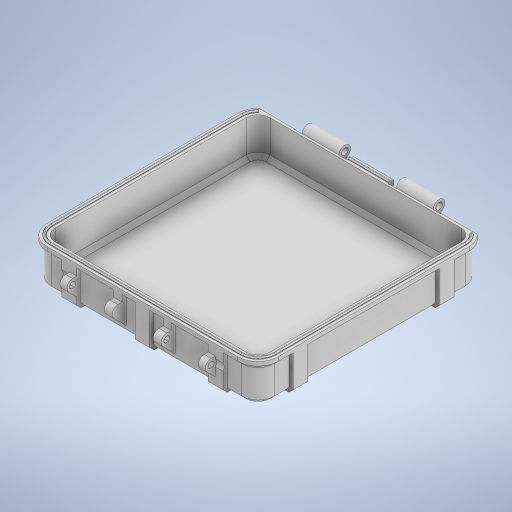
# Autodesk Inventor part: universal_box-lid
Saved by Autodesk Inventor 2024 (Build 280153000, 153)
## iProperties
Created: 2024-03-05
Part Number: universal_box-lid
Material: Všeobecné
Document SubType Name: Modeling
Designer: Simak
Density: 1 g/cm^3
Appearance: Výchozí
Author: Simak
Autodesk Inventor part; units mm, degrees
ref_plane "YZ Plane" through (0, 0, 0) normal (1, 0, 0) x (0, 1, 0)
ref_plane "XZ Plane" through (0, 0, 0) normal (0, 1, 0) x (-1, 0, 0)
sketch "velikost" plane through (0, 0, 0) normal (0, 1, 0) x (-1, 0, 0)
  line L0 (55.5, -55.5) -> (-55.5, -55.5)
  line L1 (-55.5, -55.5) -> (-55.5, 55.5)
  line L2 (-55.5, 55.5) -> (55.5, 55.5)
  line L3 (55.5, 55.5) -> (55.5, -55.5)
  line L4 (55.5, -55.5) -> (0, 0) construction
  line L5 (0, 0) -> (-55.5, -55.5) construction
  line L6 (0, 0) -> (-55.5, 55.5) construction
  dimension "d0" = 111
  dimension "d1" = 111
  constraints: 14 end point, 2 equal length, 2 parallel, 1 horizontal, 1 perpendicular
  measures "d0" distance of L0.start L0.end
  measures "d1" distance of L0.end L1.end
extrude "vyska" add sketch "velikost" along normal blind 20
fillet "Zaobleni_rohu" radius 8 4 edges at (-55.5, 10, 55.5) (55.5, 10, 55.5) (55.5, 10, -55.5) (-55.5, 10, -55.5)
shell "tloustka_sten" thickness 2 removed faces 1 at (15.8333, 20, -13.1667)
sketch "vyztuhy-velikost" plane through (0, 20, 0) normal (0, 1, 0) x (1, 0, 0)
  arc A0 (-47.5, 53.5) -> (-53.5, 47.5) centre (-47.5, 47.5) ccw projected
  line L0 (-47.5, 53.5) -> (47.5, 53.5) projected
  arc A1 (53.5, 47.5) -> (47.5, 53.5) centre (47.5, 47.5) ccw projected
  line L1 (53.5, 47.5) -> (53.5, -47.5) projected
  arc A2 (47.5, -53.5) -> (53.5, -47.5) centre (47.5, -47.5) ccw projected
  line L2 (47.5, -53.5) -> (-47.5, -53.5) projected
  arc A3 (-53.5, -47.5) -> (-47.5, -53.5) centre (-47.5, -47.5) ccw projected
  line L3 (-53.5, -47.5) -> (-53.5, 47.5) projected
  arc A4 (-47.5, 55.5) -> (-55.5, 47.5) centre (-47.5, 47.5) ccw projected
  line L4 (-55.5, 47.5) -> (-55.5, -47.5) projected
  arc A5 (-55.5, -47.5) -> (-47.5, -55.5) centre (-47.5, -47.5) ccw projected
  line L5 (-47.5, -55.5) -> (47.5, -55.5) projected
  arc A6 (47.5, -55.5) -> (55.5, -47.5) centre (47.5, -47.5) ccw projected
  line L6 (55.5, -47.5) -> (55.5, 47.5) projected
  arc A7 (55.5, 47.5) -> (47.5, 55.5) centre (47.5, 47.5) ccw projected
  line L7 (47.5, 55.5) -> (-47.5, 55.5) projected
  line L8 (-40.1, 55.5) -> (-40.1, 57.5)
  line L9 (-40.1, 57.5) -> (-32.7, 57.5)
  line L10 (-32.7, 57.5) -> (-32.7, 55.5)
  line L11 (-3.7, 55.5) -> (-3.7, 57.5)
  line L12 (-3.7, 57.5) -> (3.7, 57.5)
  line L13 (3.7, 57.5) -> (3.7, 55.5)
  line L14 (32.7, 55.5) -> (32.7, 57.5)
  line L15 (32.7, 57.5) -> (40.1, 57.5)
  line L16 (40.1, 57.5) -> (40.1, 55.5)
  line L17 (47.5, 55.5) -> (-47.5, 55.5) projected
  line L18 (-3.7, 57.5) -> (0, 55.5) construction
  line L19 (3.7, 57.5) -> (0, 55.5) construction
  line L20 (-32.7, 57.5) -> (-3.7, 57.5) construction
  line L21 (3.7, 57.5) -> (32.7, 57.5) construction
  line L22 (-40.1, 57.5) -> (-47.5, 57.5) construction
  line L23 (-47.5, 57.5) -> (-47.5, 55.5) construction
  line L24 (-53.5, 0) -> (53.5, 0)
  line L25 (0, 53.5) -> (0, -53.5)
  line L26 (47.5, -53.5) -> (-47.5, -53.5) projected
  line L27 (-55.5, -40.1) -> (-57.5, -40.1)
  line L28 (-57.5, -40.1) -> (-57.5, -32.7)
  line L29 (-57.5, -32.7) -> (-55.5, -32.7)
  line L30 (-55.5, 32.7) -> (-57.5, 32.7)
  line L31 (-57.5, 32.7) -> (-57.5, 40.1)
  line L32 (-57.5, 40.1) -> (-55.5, 40.1)
  line L33 (-57.5, -32.7) -> (-57.5, 32.7) construction
  line L34 (-57.5, -40.1) -> (-57.5, -47.5) construction
  line L35 (-57.5, -47.5) -> (-55.5, -47.5) construction
  line L36 (-55.5, 47.5) -> (-55.5, -47.5) projected
  line L37 (-57.5, 40.1) -> (-57.5, 47.5) construction
  line L38 (-57.5, 47.5) -> (-55.5, 47.5) construction
  line L39 (-55.5, 0) -> (-57.5, 32.7) construction
  line L40 (-55.5, 0) -> (-57.5, -32.7) construction
  line L41 (-40.1, -55.5) -> (-40.1, -57.5)
  line L42 (-40.1, -57.5) -> (-32.7, -57.5)
  line L43 (-32.7, -57.5) -> (-32.7, -55.5)
  line L44 (-3.7, -55.5) -> (-3.7, -57.5)
  line L45 (-3.7, -57.5) -> (3.7, -57.5)
  line L46 (3.7, -57.5) -> (3.7, -55.5)
  line L47 (32.7, -55.5) -> (32.7, -57.5)
  line L48 (32.7, -57.5) -> (40.1, -57.5)
  line L49 (40.1, -57.5) -> (40.1, -55.5)
  line L50 (47.5, -55.5) -> (-47.5, -55.5)
  line L51 (-3.7, -57.5) -> (0, -55.5) construction
  line L52 (3.7, -57.5) -> (0, -55.5) construction
  line L53 (-32.7, -57.5) -> (-3.7, -57.5) construction
  line L54 (3.7, -57.5) -> (32.7, -57.5) construction
  line L55 (-40.1, -57.5) -> (-47.5, -57.5) construction
  line L56 (-47.5, -57.5) -> (-47.5, -55.5) construction
  line L57 (55.5, 47.5) -> (55.5, -47.5)
  line L58 (57.5, -32.7) -> (57.5, 32.7) construction
  line L59 (55.5, -40.1) -> (57.5, -40.1)
  line L60 (57.5, -40.1) -> (57.5, -47.5) construction
  line L61 (57.5, -32.7) -> (55.5, -32.7)
  line L62 (57.5, -47.5) -> (55.5, -47.5) construction
  line L63 (57.5, -40.1) -> (57.5, -32.7)
  line L64 (57.5, 32.7) -> (57.5, 40.1)
  line L65 (57.5, 40.1) -> (55.5, 40.1)
  line L66 (55.5, 32.7) -> (57.5, 32.7)
  line L67 (55.5, 47.5) -> (55.5, -47.5)
  line L68 (57.5, 40.1) -> (57.5, 47.5) construction
  line L69 (57.5, 47.5) -> (55.5, 47.5) construction
  line L70 (55.5, 0) -> (57.5, 32.7) construction
  line L71 (55.5, 0) -> (57.5, -32.7) construction
  point P0 (0, 0)
  point P1 (55.5, 40.1)
  point P2 (55.5, 32.7)
  point P3 (55.5, -32.7)
  point P4 (55.5, -40.1)
  point P5 (40.1, -55.5)
  point P6 (32.7, -55.5)
  point P7 (3.7, -55.5)
  point P8 (-3.7, -55.5)
  point P9 (-32.7, -55.5)
  point P10 (-40.1, -55.5)
  point P11 (-55.5, -40.1)
  point P12 (-55.5, 32.7)
  point P13 (-55.5, 40.1)
  dimension "d6" = 2
  dimension "d7" = 7.4
  dimension "d8" = 2
  constraints: 120 end point, 25 symmetric about line, 20 point on line, 14 equal length, 11 perpendicular, 5 midpoint, 5 vertical, 2 horizontal, 5 other
  measures "d6" distance of L9.end L10.end
  measures "d7" distance of L11.end L12.end
  measures "d8" distance of L33.start L29.end
extrude "vyztuhy" add sketch "vyztuhy-velikost" against normal up to surface (20 mm away) contours L8 L9 L10 L7 | L4 L30 L31 L32 | L11 L12 L13 L7 | L4 L27 L28 L29 | L14 L15 L16 L7 | L5 L43 L42 L41 | L65 L64 L66 L6 | L5 L46 L45 L44 | L61 L63 L59 L6 | L5 L49 L48 L47
chamfer "Zkoseni_spodku" distance 2 angle 45 36 edges at (-18.2, 0, 55.5) (18.2, 0, 55.5) (0, 0, 57.5) (36.4, 0, 57.5) (43.8, 0, 55.5) (53.1569, 0, 53.1569) (55.5, 0, 43.8) (57.5, 0, 36.4) (55.5, 0, 0) (57.5, 0, -36.4) (53.1569, 0, -53.1569) (43.8, 0, -55.5) (55.5, 0, -43.8) (36.4, 0, -57.5) (18.2, 0, -55.5) (0, 0, -57.5) (-18.2, 0, -55.5) (-36.4, 0, -57.5) (-43.8, 0, -55.5) (-53.1569, 0, -53.1569) (-55.5, 0, -43.8) (-57.5, 0, -36.4) (-55.5, 0, 0) (-57.5, 0, 36.4) (-55.5, 0, 43.8) (-53.1569, 0, 53.1569) (-43.8, 0, 55.5) (-36.4, 0, 57.5) (-53.5, 2, 0) (-51.7426, 2, 51.7426) (0, 2, 53.5) (51.7426, 2, 51.7426) (53.5, 2, 0) (51.7426, 2, -51.7426) (0, 2, -53.5) (-51.7426, 2, -51.7426)
sketch "Náčrt4" plane through (40.1, 20, -55.5) normal (1, 0, 0) x (0, 0, -1)
  line L0 (-2, 0) -> (-2, -16) projected
  line L1 (2, 0) -> (2, -18) projected
  line L2 (-8, 0) -> (0, 0) projected
  line L3 (-0.7, 0) -> (-0.7, 0.3)
  line L4 (-0.7, 0.3) -> (0.7, 0.3)
  line L5 (0.7, 0.3) -> (0.7, 0)
  line L6 (-0.7, 0.3) -> (-2, 0.3) construction
  line L7 (0.7, 0.3) -> (2, 0.3) construction
  line L8 (2, 0) -> (0, 0) projected
  line L9 (2, -4) -> (-2, -4)
  line L10 (-0.6, 0.3) -> (-0.1631, 0.9157)
  arc A0 (0.1631, 0.9157) -> (-0.1631, 0.9157) centre (0, 0.8) ccw
  line L11 (0.1631, 0.9157) -> (0.6, 0.3)
  point P0 (-55.5, -20)
  point P1 (0, 0.3)
  point P2 (0, 1)
  dimension "d16" = 1.4
  dimension "d71" = 4
  dimension "d72" = 0.3
  dimension "d75" = 1
  dimension "d76" = 0.2
  dimension "d77" = 0.6
  constraints: 16 end point, 9 point on line, 5 perpendicular, 3 point on circle, 3 vertical alignment, 2 equal length, 2 tangent, 1 centre point, 1 midpoint
  measures "d16" distance of L3.end L4.end
  measures "d71" distance between parallel lines of L9 L8
  measures "d72" distance between parallel lines of L8 L4
  measures "d75" distance from line of L8 point (0, 1)
  measures "d76" radius of A0
  measures "d77" horizontal distance of L11.end A0.centre
sketch "Náčrt3" plane through (0, 20, 0) normal (0, 1, 0) x (1, 0, 0)
  arc A0 (-47.5, 53.5) -> (-53.5, 47.5) centre (-47.5, 47.5) ccw projected
  line L0 (-47.5, 53.5) -> (47.5, 53.5) projected
  arc A1 (53.5, 47.5) -> (47.5, 53.5) centre (47.5, 47.5) ccw projected
  line L1 (53.5, 47.5) -> (53.5, -47.5) projected
  arc A2 (47.5, -53.5) -> (53.5, -47.5) centre (47.5, -47.5) ccw projected
  line L2 (47.5, -53.5) -> (-47.5, -53.5) projected
  arc A3 (-53.5, -47.5) -> (-47.5, -53.5) centre (-47.5, -47.5) ccw projected
  line L3 (-53.5, -47.5) -> (-53.5, 47.5) projected
  arc A4 (-47.5, 55.5) -> (-55.5, 47.5) centre (-47.5, 47.5) ccw projected
  line L4 (-55.5, 47.5) -> (-55.5, 40.1) projected
  line L5 (-57.5, 32.7) -> (-55.5, 32.7) projected
  line L6 (-55.5, 32.7) -> (-55.5, -32.7) projected
  line L7 (-55.5, -32.7) -> (-57.5, -32.7) projected
  line L8 (-57.5, -32.7) -> (-57.5, -40.1) projected
  arc A5 (-55.5, -47.5) -> (-47.5, -55.5) centre (-47.5, -47.5) ccw projected
  line L9 (-47.5, -55.5) -> (-40.1, -55.5) projected
  line L10 (-40.1, -55.5) -> (-40.1, -57.5) projected
  line L11 (-40.1, -57.5) -> (-32.7, -57.5) projected
  line L12 (-32.7, -57.5) -> (-32.7, -55.5) projected
  line L13 (-32.7, -55.5) -> (-3.7, -55.5) projected
  line L14 (-3.7, -55.5) -> (-3.7, -57.5) projected
  line L15 (-3.7, -57.5) -> (3.7, -57.5) projected
  line L16 (3.7, -57.5) -> (3.7, -55.5) projected
  line L17 (3.7, -55.5) -> (32.7, -55.5) projected
  line L18 (32.7, -55.5) -> (32.7, -57.5) projected
  line L19 (32.7, -57.5) -> (40.1, -57.5) projected
  line L20 (40.1, -57.5) -> (40.1, -55.5) projected
  line L21 (40.1, -55.5) -> (47.5, -55.5) projected
  arc A6 (47.5, -55.5) -> (55.5, -47.5) centre (47.5, -47.5) ccw projected
  line L22 (55.5, -47.5) -> (55.5, -40.1) projected
  line L23 (57.5, -32.7) -> (55.5, -32.7) projected
  line L24 (55.5, -32.7) -> (55.5, 32.7) projected
  line L25 (55.5, 32.7) -> (57.5, 32.7) projected
  line L26 (57.5, 32.7) -> (57.5, 40.1) projected
  arc A7 (55.5, 47.5) -> (47.5, 55.5) centre (47.5, 47.5) ccw projected
  line L27 (47.5, 55.5) -> (40.1, 55.5) projected
  line L28 (40.1, 55.5) -> (40.1, 57.5) projected
  line L29 (40.1, 57.5) -> (32.7, 57.5) projected
  line L30 (32.7, 57.5) -> (32.7, 55.5) projected
  line L31 (32.7, 55.5) -> (3.7, 55.5) projected
  line L32 (3.7, 55.5) -> (3.7, 57.5) projected
  line L33 (3.7, 57.5) -> (-3.7, 57.5) projected
  line L34 (-3.7, 57.5) -> (-3.7, 55.5) projected
  line L35 (-3.7, 55.5) -> (-32.7, 55.5) projected
  line L36 (-32.7, 55.5) -> (-32.7, 57.5) projected
  line L37 (-32.7, 57.5) -> (-40.1, 57.5) projected
  line L38 (-40.1, 57.5) -> (-40.1, 55.5) projected
  line L39 (-40.1, 55.5) -> (-47.5, 55.5) projected
  line L40 (-55.5, 40.1) -> (-57.5, 40.1) projected
  line L41 (-57.5, 40.1) -> (-57.5, 32.7) projected
  line L42 (-57.5, -40.1) -> (-55.5, -40.1) projected
  line L43 (-55.5, -40.1) -> (-55.5, -47.5) projected
  line L44 (55.5, -40.1) -> (57.5, -40.1) projected
  line L45 (57.5, -40.1) -> (57.5, -32.7) projected
  line L46 (57.5, 40.1) -> (55.5, 40.1) projected
  line L47 (55.5, 40.1) -> (55.5, 47.5) projected
  point P0 (0, 0)
sweep "tesnici_drazka" add profiles "Náčrt4" path "Náčrt3" path curves L0 A0 L3 A3 L2 A2 L1 A1
chamfer "tesnici_drazka-zkoseni" distance 2 angle 45 18 edges at (54.5711, 16, -54.5711) (43.8, 16, -57.5) (57.5, 16, -43.8) (18.2, 16, -57.5) (-18.2, 16, -57.5) (57.5, 16, 0) (57.5, 16, 43.8) (54.5711, 16, 54.5711) (43.8, 16, 57.5) (-54.5711, 16, -54.5711) (-57.5, 16, -43.8) (-43.8, 16, -57.5) (-57.5, 16, 0) (-54.5711, 16, 54.5711) (-43.8, 16, 57.5) (-57.5, 16, 43.8) (18.2, 16, 57.5) (-18.2, 16, 57.5)
sketch "Náčrt16" plane through (32.7, 0, -55.5) normal (-1, 0, 0) x (0, 0, 1)
  line L0 (-2, 18) -> (-2, 2) projected
  line L1 (0, 0) -> (-2, 2) projected
  line L2 (2, 0) -> (0, 0) projected
  line L3 (0, 2) -> (2, 0) projected
  line L4 (0, 16) -> (0, 2) projected
  line L5 (-2, 18) -> (0, 16) projected
  line L6 (8, 20) -> (-2, 20) projected
  circle A0 centre (-2, 20) radius 1.65
  circle A1 centre (-2, 20) radius 2.7
  circle A2 centre (-2, 20) radius 2.875
  circle A3 centre (-2, 20) radius 3.025
  line L7 (0, 13.9341) -> (-4.0329, 17.9671)
  point P0 (55.5, 0)
  point P1 (0.875, 20)
  point P2 (-1.1092, 17.1092)
  point P3 (1.025, 20)
  point P4 (-3.3677, 17.3019)
  point P5 (-2, 15.9341)
  point P6 (-2, 16.975)
  dimension "d148" = 5.75
  dimension "d147" = 3.3
  dimension "d149" = 5.4
  dimension "d150" = 0.15
  dimension "d151" = 45
  constraints: 3 centre point, 3 coincident, 2 end point, 1 point on line, 4 other
  measures "d147" diameter of A0
  measures "d149" diameter of A1
  measures "d151" angle of L4 L7
extrude "Vysunutí23" cut sketch "Náčrt16" along normal blind 22.65 and the other way blind 3.65 contours L5 A1 L0 | L0 A1 L5 | A1 L5 A2 L0 | L0 A2 L6 A1 | A1 L6 A2 L5 | A2 L5 A3 L0 | L0 A3 L7 A2 | A2 L6 A3 L5 | L7 A3 L6 A2 | A0
extrude "Vysunutí24" cut sketch "Náčrt16" against normal through all contours L5 A1 L0 | L0 A1 L5 | A0
extrude "Vysunutí25" add sketch "Náčrt16" along normal blind 18.4 contours L5 A1 L0 | L0 A1 L5 | A1 L5 A2 L0 | L0 A2 L6 A1 | A1 L6 A2 L5 | A2 L5 A3 L0 | L0 A3 L7 A2 | A2 L6 A3 L5 | A3 L5 L4 L7 L0 | L0 L7 A3
extrude "Vysunutí26" cut sketch "Náčrt16" along normal blind 0.1 contours L5 A1 L0 | L0 A1 L5 | A1 L5 A2 L0 | L0 A2 L6 A1 | A1 L6 A2 L5 | A2 L5 A3 L0 | L0 A3 L7 A2 | A2 L6 A3 L5 | L0 L7 A3 | L7 A3 L6 A2 | A0
sketch "Náčrt17" plane through (0, 20, 0) normal (0, 1, 0) x (1, 0, 0)
  arc A0 (-47.5, 53.5) -> (-53.5, 47.5) centre (-47.5, 47.5) ccw projected
  line L0 (-47.5, 53.5) -> (47.5, 53.5) projected
  arc A1 (53.5, 47.5) -> (47.5, 53.5) centre (47.5, 47.5) ccw projected
  line L1 (53.5, 47.5) -> (53.5, -47.5) projected
  arc A2 (47.5, -53.5) -> (53.5, -47.5) centre (47.5, -47.5) ccw projected
  line L2 (47.5, -53.5) -> (-47.5, -53.5) projected
  arc A3 (-53.5, -47.5) -> (-47.5, -53.5) centre (-47.5, -47.5) ccw projected
  line L3 (-53.5, -47.5) -> (-53.5, 47.5) projected
  arc A4 (-47.5, 54.8) -> (-54.8, 47.5) centre (-47.5, 47.5) ccw projected
  line L4 (-54.8, 47.5) -> (-54.8, -47.5) projected
  arc A5 (-54.8, -47.5) -> (-47.5, -54.8) centre (-47.5, -47.5) ccw projected
  line L5 (-47.5, -54.8) -> (47.5, -54.8) projected
  arc A6 (47.5, -54.8) -> (54.8, -47.5) centre (47.5, -47.5) ccw projected
  line L6 (54.8, -47.5) -> (54.8, 47.5) projected
  arc A7 (54.8, 47.5) -> (47.5, 54.8) centre (47.5, 47.5) ccw projected
  line L7 (47.5, 54.8) -> (36.35, 54.8) projected
  line L8 (36.35, 54.8) -> (36.35, 54.475) projected
  line L9 (36.35, 54.475) -> (32.6, 54.475) projected
  line L10 (32.6, 54.475) -> (32.6, 54.625) projected
  line L11 (32.6, 54.625) -> (14.3, 54.625) projected
  line L12 (14.3, 54.475) -> (14.3, 54.625) projected
  line L13 (14.3, 54.475) -> (10.05, 54.475) projected
  line L14 (10.05, 54.475) -> (10.05, 54.8) projected
  line L15 (10.05, 54.8) -> (-47.5, 54.8) projected
  arc A8 (-47.5, 57.5) -> (-57.5, 47.5) centre (-47.5, 47.5) ccw projected
  line L16 (-57.5, 47.5) -> (-57.5, -47.5) projected
  arc A9 (-57.5, -47.5) -> (-47.5, -57.5) centre (-47.5, -47.5) ccw projected
  line L17 (-47.5, -57.5) -> (47.5, -57.5) projected
  arc A10 (47.5, -57.5) -> (57.5, -47.5) centre (47.5, -47.5) ccw projected
  line L18 (57.5, -47.5) -> (57.5, 47.5) projected
  arc A11 (57.5, 47.5) -> (54.3345, 54.8) centre (47.5, 47.5) ccw projected
  line L19 (54.3345, 54.8) -> (52.2329, 54.8) projected
  arc A12 (56.2, 47.5) -> (52.2329, 54.8) centre (47.5, 47.5) ccw projected
  line L20 (56.2, -47.5) -> (56.2, 47.5) projected
  arc A13 (47.5, -56.2) -> (56.2, -47.5) centre (47.5, -47.5) ccw projected
  line L21 (-47.5, -56.2) -> (47.5, -56.2) projected
  arc A14 (-56.2, -47.5) -> (-47.5, -56.2) centre (-47.5, -47.5) ccw projected
  line L22 (-56.2, 47.5) -> (-56.2, -47.5) projected
  arc A15 (-47.5, 56.2) -> (-56.2, 47.5) centre (-47.5, 47.5) ccw projected
  spline S0 degree 8 poles (47.5, 56.8737) (48.0163, 56.8737) (48.5323, 56.8475) (49.0473, 56.7951) (49.5603, 56.7176) (50.0703, 56.6177) (50.5764, 56.4985) (51.0774, 56.3641) (51.7861, 56.1565) (51.9987, 56.092) (52.21, 56.0258) (52.4199, 55.9585) (52.6283, 55.8905) (52.8351, 55.8221) (53.0401, 55.7539) (53.2432, 55.6863) knots 0 0 0 0 0 0 0 0 0 0.698385 0.698385 0.698385 0.698385 0.698385 0.698385 0.698385 1 1 1 1 1 1 1 1 1 projected
  line L23 (40.1, 56.8737) -> (47.5, 56.8737) projected
  line L24 (40.1, 57.5) -> (40.1, 56.8737) projected
  line L25 (36.35, 57.5) -> (40.1, 57.5) projected
  line L26 (36.35, 54.8) -> (36.35, 57.5) projected
  line L27 (47.5, 54.8) -> (36.35, 54.8) projected
  line L28 (36.35, 54.8167) -> (36.35, 54.8) projected
  line L29 (48.6071, 54.8167) -> (36.35, 54.8167) projected
  line L30 (52.207, 54.8167) -> (52.0195, 54.8167) projected
  line L31 (54.3345, 54.8) -> (52.2329, 54.8) projected
  spline S1 degree 6 poles (53.2432, 55.6863) (53.3272, 55.6273) (53.4089, 55.5685) (53.4878, 55.5102) (53.5637, 55.4527) (53.6363, 55.3964) (53.7493, 55.307) (53.7917, 55.273) (53.8326, 55.2397) (53.8719, 55.2073) (53.9096, 55.1759) (53.9724, 55.1229) (53.9985, 55.1008) (54.0235, 55.0793) (54.0475, 55.0586) (54.0703, 55.0387) (54.1714, 54.9501) (54.2361, 54.8916) (54.2852, 54.8462) (54.318, 54.8154) (54.3345, 54.8) (54.3345, 54.8) knots 0 0 0 0 0 0 0 0.258993 0.258993 0.258993 0.258993 0.258993 0.423699 0.423699 0.423699 0.423699 0.423699 0.547895 0.547895 0.547895 0.547895 0.547895 1 1 1 1 1 1 1 projected
  line L32 (36.35, 54.475) -> (36.35, 53.5)
  line L33 (47.5, 47.5) -> (53.5, 53.8)
  line L34 (10.05, 56.2) -> (-47.5, 56.2) projected
  line L35 (10.05, 56.2) -> (10.05, 57.5) projected
  line L36 (10.05, 57.5) -> (-47.5, 57.5) projected
  point P0 (0, 0)
  point P1 (36.35, 54.8167)
  point P2 (52.5345, 52.7862)
  point P3 (46.7329, 24.3)
  point P4 (54.3345, 54.8)
  point P5 (51.7329, 54.3)
  dimension "d162" = 1
  constraints: 4 end point, 1 horizontal alignment, 1 perpendicular, 1 point on circle, 1 point on line, 5 other
  measures "d162" distance from line of L19 L33.end
extrude "Vysunutí27" cut sketch "Náčrt17" along normal through all contours L26 L25 L24 L23 S0 S1 L19 A12 L33 A7 L7
sketch "Náčrt18" plane through (32.6, 0, -55.5) normal (1, 0, 0) x (0, 0, -1)
  line L0 (4.0329, 17.9671) -> (2, 15.9341) projected
  arc A0 (4.0329, 17.9671) -> (-0.875, 20) centre (2, 20) ccw projected
  line L1 (-1.025, 20) -> (-0.875, 20) projected
  arc A1 (-1.025, 20) -> (2, 16.975) centre (2, 20) ccw projected
  line L2 (2, 15.9341) -> (2, 16.975) projected
  circle A2 centre (2, 20) radius 1.65 projected
  circle A3 centre (2, 20) radius 2.875
  line L3 (-0.139, 17.861) -> (2, 15.722)
  line L4 (2, 18) -> (2, 2) projected
  arc A4 (-1.025, 20) -> (1.1092, 17.1092) centre (2, 20) ccw projected
  point P0 (-55.5, 0)
  point P1 (-0.139, 17.861)
  dimension "d165" = 45
  constraints: 3 point on circle, 2 end point, 1 coincident, 1 horizontal alignment, 1 point on line, 1 tangent, 2 other
  measures "d165" angle of L4 L3
extrude "Vysunutí28" cut sketch "Náčrt18" along normal up to surface (3.75 mm away) contours L4 L3 A1 L2
sketch "Náčrt19" plane through (14.3, 0, -55.5) normal (-1, 0, 0) x (0, 0, 1)
  line L0 (-4.0329, 17.9671) -> (-1.8939, 15.8281) projected
  arc A0 (0.875, 20) -> (-4.0329, 17.9671) centre (-2, 20) ccw projected
  line L1 (1.025, 20) -> (0.875, 20) projected
  arc A1 (0.139, 17.861) -> (1.025, 20) centre (-2, 20) ccw projected
  line L2 (0.139, 17.861) -> (-1.8939, 15.8281) projected
  circle A2 centre (-2, 20) radius 1.65 projected
  point P0 (55.5, 0)
extrude "Vysunutí29" cut sketch "Náčrt19" along normal up to surface (4.25 mm away)
mirror "Zrcadlit4" about plane through (0, 0, 0) normal (1, 0, 0) of "Vysunutí23", "Vysunutí24", "Vysunutí25", "Vysunutí26", "Vysunutí27", "Vysunutí28", "Vysunutí29"
sketch "latch-main_nacrt" plane through (32.7, 0, 53.5) normal (-1, 0, 0) x (0, 0, 1)
  line L0 (4, 18) -> (4, 2) projected
  line L1 (2, 0) -> (4, 2) projected
  line L2 (0, 0) -> (2, 0) projected
  line L3 (2, 2) -> (0, 0) projected
  line L4 (2, 16) -> (2, 2) projected
  line L5 (4, 18) -> (2, 16) projected
  line L6 (4, 20) -> (-6, 20) projected
  line L7 (2.7, 20.3) -> (-6, 20.3) projected
  line L8 (1.25, 23) -> (1.25, 25) projected
  line L9 (2.7, 20.3) -> (2.7, 20) projected
  line L10 (4, 20) -> (4, 18) projected
  circle A0 centre (6.05, 11.8) radius 1.55
  line L11 (5.3, 10.4435) -> (5.3, 10.6)
  line L12 (5.3, 10.6) -> (6.8, 10.6)
  line L13 (6.8, 10.6) -> (6.8, 10.4435)
  circle A1 centre (6.05, 11.8) radius 2.875
  line L14 (6.05, 14.675) -> (2, 14.675)
  line L15 (2, 3.6841) -> (8.0829, 9.7671)
  circle A2 centre (6.05, 11.8) radius 2.7
  point P0 (-53.5, 0)
  point P1 (4, 13.8157)
  point P2 (4, 9.7843)
  dimension "d52" = 3.1
  dimension "d53" = 8.2
  dimension "d54" = 4.05
  dimension "d55" = 2.75
  dimension "d56" = 1.5
  dimension "d57" = 5.75
  dimension "d58" = 45
  dimension "d63" = 5.4
  constraints: 10 end point, 4 point on circle, 3 centre point, 3 perpendicular, 2 coincident, 2 point on line, 2 tangent, 1 parallel, 1 vertical, 2 other
  measures "d52" diameter of A0
  measures "d54" distance from line of L4 A0.centre
  measures "d56" distance of L11.end L12.end
  measures "d57" diameter of A1
  measures "d58" angle of L4 L15
  measures "d63" diameter of A2
extrude "Vysunutí14" cut sketch "latch-main_nacrt" against normal up to next contours A2 L0 | L0 A2
extrude "Vysunutí12" add sketch "latch-main_nacrt" against normal blind 3.5 contours L14 A1 L0 | L0 A1 L15 L4 L14 | A1 L0 A2 | L0 A2 A1 | A2 L0 | L0 A2 | A1 L15 L0 | L11 L12 L13 A0 picked at (5.9979, 10.486)
ref_plane "Pracovní rovina3" through (14.2, 0, 53.5) normal (-1, 0, 0) x (0, 0, 1)
sketch "Náčrt10" plane through (14.2, 0, 53.5) normal (-1, 0, 0) x (0, 0, 1)
  arc A0 (6.8, 10.4435) -> (5.3, 10.4435) centre (6.05, 11.8) ccw projected
  line L0 (6.8, 10.4435) -> (6.8, 10.6) projected
  line L1 (6.8, 10.6) -> (5.3, 10.6) projected
  line L2 (5.3, 10.6) -> (5.3, 10.4435) projected
  line L3 (4, 5.6841) -> (8.0829, 9.7671) projected
  arc A1 (8.0829, 9.7671) -> (6.05, 14.675) centre (6.05, 11.8) ccw projected
  line L4 (6.05, 14.675) -> (4, 14.675) projected
  line L5 (4, 18) -> (4, 14.675) projected
  line L6 (2, 16) -> (4, 18) projected
  line L7 (2, 2) -> (2, 16) projected
  line L8 (0, 0) -> (2, 2) projected
  line L9 (2, 0) -> (0, 0) projected
  line L10 (4, 2) -> (2, 0) projected
  line L11 (4, 5.6841) -> (4, 2) projected
  line L12 (4, 14.675) -> (2, 14.675)
  line L13 (4, 5.6841) -> (2, 3.6841)
  line L14 (4, 14.675) -> (2, 16)
  point P0 (-53.5, 0)
  constraints: 6 end point, 2 collinear, 2 point on line
extrude "Vysunutí15" add sketch "Náčrt10" along normal blind 4 contours L13 L7 L12 L4 A1 L3 | L7 L14 L12 | L14 L6 L5
sketch "Náčrt12" plane through (10.2, 0, 53.5) normal (-1, 0, 0) x (0, 0, 1)
  line L0 (2, 3.6841) -> (8.0829, 9.7671) projected
  arc A0 (8.0829, 9.7671) -> (6.05, 14.675) centre (6.05, 11.8) ccw projected
  line L1 (6.05, 14.675) -> (4, 14.675) projected
  line L2 (6.8, 10.6) -> (5.3, 10.6) projected
  line L3 (5.3, 10.6) -> (5.3, 10.4435) projected
  arc A1 (6.8, 10.4435) -> (5.3, 10.4435) centre (6.05, 11.8) ccw projected
  line L4 (6.8, 10.4435) -> (6.8, 10.6) projected
  line L5 (4, 14.675) -> (4, 18) projected
  line L6 (2, 16) -> (4, 18) projected
  line L7 (2, 3.6841) -> (2, 16) projected
  point P0 (-53.5, 0)
extrude "Vysunutí16" add sketch "Náčrt12" against normal blind 0.5 contours L2 L3 A1 L4
mirror "latch-zrcadleni" about plane through (0, 0, 0) normal (1, 0, 0) of "Vysunutí16", "Vysunutí14", "Vysunutí12", "Vysunutí15"
fillet "Zaoblení2" radius 1 8 edges at (-43.8, 17.3736, -56.8737) (-50.4352, 17.4845, -56.519) (-54.0393, 18.8323, -55.0656) (-38.225, 17.3, -57.5) (38.225, 17.3, -57.5) (50.4352, 17.4845, -56.519) (43.8, 17.3736, -56.8737) (54.0393, 18.8323, -55.0656)
ref_plane "Pracovní rovina4" through (-14.2, 0, 53.5) normal (-1, 0, 0) x (0, 0, 1)
